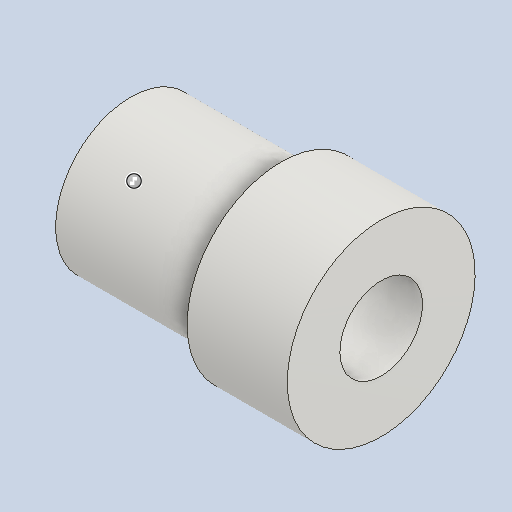
# Autodesk Inventor part: Wał
Saved by Autodesk Inventor 2023 (Build 270158000, 158)
## iProperties
Created: 2023-05-12
Part Number: Wał
Material: Steel
Document SubType Name: Modeling
Designer: krzys
Density: 1 g/cm^3
Appearance: Steel
CustomPartVersion: 1
Author: krzys
Length: 20,000 mm
Autodesk Inventor part; units mm, degrees
ref_plane "Płaszczyzna początkowa" through (0, 0, 0) normal (1, 0, 0) x (0, 1, 0)
ref_plane "XZ Plane" through (0, 0, 0) normal (0, 1, 0) x (-1, 0, 0)
ref_plane "XY Plane" through (0, 0, 0) normal (0, 0, 1) x (1, 0, 0)
sketch "Szkic główny" plane through (0, 0, 0) normal (0, 0, 1) x (1, 0, 0)
  line L0 (0, 0) -> (20, 0)
  line L1 (0, 0) -> (0, 6)
  line L2 (0, 6) -> (12, 6)
  line L3 (12, 6) -> (12, 7.5)
  line L4 (20, 7.5) -> (20, 0)
  line L5 (12, 7.5) -> (20, 7.5)
  dimension "d11" = 12
  dimension "d12" = 15
  constraints: 12 end point, 4 horizontal, 3 vertical
  measures "d11" diameter of L2 L0
  measures "d12" diameter of L5 L0
revolve "Obrót1" add sketch "Szkic główny" angle 360 about axis through (0, 0, 0) along (1, 0, 0)
sketch "Szkic3" plane through (0, 0, 0) normal (-1, 0, 0) x (0, 0, 1)
  point P0 (0, 0)
hole "Otwór1" at (0, 0, 0) direction (1, 0, 0) diameter 6.6 end through all
equation "\"Length\" = 20"
